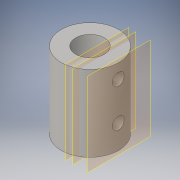
# Autodesk Inventor part: Motor Coupler
Saved by Autodesk Inventor 2016 (Build 200138000, 138)
## iProperties
Created: 2016-04-23
Part Number: Motor Coupler
Material: ABS Plastic
Document SubType Name: Modeling
Designer: rubenjm
Density: 1.06 g/cm^3
Appearance: Smooth - White
Author: rubenjm
Autodesk Inventor part; units mm, degrees
ref_plane "XZ Plane" through (0, 0, 0) normal (0, 1, 0) x (-1, 0, 0)
ref_plane "XY Plane" through (0, 0, 0) normal (0, 0, 1) x (1, 0, 0)
sketch "Sketch1" plane through (0, 0, 0) normal (0, 1, 0) x (-1, 0, 0)
  circle A0 centre (0, 0) radius 12.7
  dimension "d0" = 25.4
  constraints: 1 centre point, 1 coincident
  measures "d0" diameter of A0
extrude "Extrusion1" add sketch "Sketch1" along normal blind 33.7058
sketch "Sketch2" plane through (0, 0, 0) normal (0, -1, 0) x (1, 0, 0)
  circle A0 centre (0, 0) radius 3.175
  dimension "d3" = 6.35
  constraints: 1 centre point, 1 coincident
  measures "d3" diameter of A0
extrude "Extrusion2" cut sketch "Sketch2" against normal blind 21.0058
sketch "Sketch3" plane through (0, 33.7058, 0) normal (0, 1, 0) x (1, 0, 0)
  circle A0 centre (0, 0) radius 6.35
  dimension "d6" = 12.7
  constraints: 1 centre point, 1 coincident
  measures "d6" diameter of A0
extrude "Extrusion3" cut sketch "Sketch3" against normal blind 12.7
ref_plane "Work Plane1" through (3.175, 0, 0) normal (1, 0, 0) x (0, 1, 0)
sketch "Sketch4" plane through (3.175, 0, 0) normal (1, 0, 0) x (0, 1, 0)
  line L0 (0, 0) -> (21.0058, 0) construction
  line L1 (21.0058, -3.175) -> (21.0058, 3.175) construction
  circle A0 centre (10.5029, 0) radius 2.55
  dimension "d10" = 5.1
  constraints: 2 end point, 2 midpoint, 1 centre point
  measures "d10" diameter of A0
ref_plane "Work Plane2" through (6.35, 0, 0) normal (1, 0, 0) x (0, 1, 0)
sketch "Sketch5" plane through (6.35, 0, 0) normal (1, 0, 0) x (0, 1, 0)
  line L0 (33.4751, 0) -> (21.0058, 0) construction
  line L1 (21.0058, -3.175) -> (21.0058, 3.175) construction
  circle A0 centre (27.2404, 0) radius 2.55
  point P0 (0, 0)
  dimension "d12" = 5.1
  constraints: 2 end point, 2 midpoint, 1 centre point
  measures "d12" diameter of A0
ref_plane "Work Plane3" through (12.7, 0, 0) normal (1, 0, 0) x (0, 1, 0)
sketch "Sketch6" plane through (12.7, 0, 0) normal (1, 0, 0) x (0, 1, 0)
  line L0 (21.0058, -3.175) -> (21.0058, 3.175) construction
  line L1 (21.0058, 0) -> (0, 0) construction
  circle A0 centre (10.5029, 0) radius 2.65
  dimension "d14" = 5.3
  constraints: 2 end point, 2 midpoint, 1 centre point, 1 horizontal
  measures "d14" diameter of A0
sketch "Sketch7" plane through (12.7, 0, 0) normal (1, 0, 0) x (0, 1, 0)
  line L0 (21.0058, -3.175) -> (21.0058, 3.175) construction
  line L1 (21.0058, 0) -> (33.7221, 0) construction
  circle A0 centre (27.364, 0) radius 2.65
  point P0 (0, 0)
  dimension "d15" = 5.3
  constraints: 2 end point, 2 midpoint, 1 centre point, 1 horizontal
  measures "d15" diameter of A0
loft "Loft1" cut profiles "Sketch4", "Sketch6"
loft "Loft2" cut profiles "Sketch5", "Sketch7"
body "Solid1"
